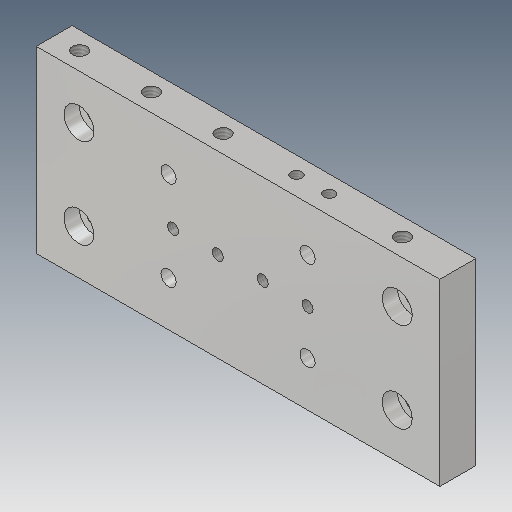
# Autodesk Inventor part: XcolBracket
Saved by Autodesk Inventor 2019 (Build 230136000, 136)
## iProperties
Created: 2018-10-03
Part Number: XcolBracket
Material: Aluminum 6061-AHC
Document SubType Name: Modeling
Designer: LillaHunden
Mass: 74.1972 g
Surface Area: 104.645 cm^2
Volume: 27.4804 cm^3
Density: 2.7 g/cm^3
Appearance: Aluminum - Dark
Author: LillaHunden
Autodesk Inventor part; units mm, degrees
ref_plane "YZ Plane" through (0, 0, 0) normal (1, 0, 0) x (0, 1, 0)
ref_plane "XZ Plane" through (0, 0, 0) normal (0, 1, 0) x (-1, 0, 0)
ref_plane "XY Plane" through (0, 0, 0) normal (0, 0, 1) x (1, 0, 0)
sketch "Sketch1" plane through (0, 0, 0) normal (0, 0, 1) x (1, 0, 0)
  line L0 (22.4756, 17.0801) -> (-67.5244, 17.0801)
  line L1 (-67.5244, 17.0801) -> (-67.5244, -22.9199)
  line L2 (-67.5244, -22.9199) -> (22.4756, -22.9199)
  line L3 (22.4756, -22.9199) -> (22.4756, 17.0801)
  point P0 (0, 0)
  dimension "d0" = 90
  dimension "d53" = 40
  constraints: 8 end point, 2 parallel, 1 horizontal, 1 perpendicular
  measures "d0" distance of L2.end L1.end
  measures "d53" distance of L0.end L1.end
extrude "Extrusion1" add sketch "Sketch1" along normal blind 8
sketch "Sketch2" plane through (0, 0, 8) normal (0, 0, 1) x (1, 0, 0)
  point P0 (12.9756, 7.0801)
  point P1 (12.9756, -12.9199)
  point P2 (-58.0244, 7.0801)
  point P3 (-58.0244, -12.9199)
hole "Hole1" at (12.9756, 7.0801, 8) at (12.9756, -12.9199, 8) at (-58.0244, 7.0801, 8) at (-58.0244, -12.9199, 8) direction (0, 0, -1) diameter 3.4 depth 8 counterbore diameter 6.7 counterbore depth 3.4
sketch "Sketch3" plane through (-67.5244, 17.0801, 0) normal (0, 1, 0) x (1, 0, 0)
  point P0 (61.1484, -12.9831)
  point P1 (53.8516, -12.9831)
  point P2 (61.15, -3.819)
  point P3 (53.85, -3.819)
hole "Hole3" at (-6.376, 17.0801, 12.9831) at (-13.6728, 17.0801, 12.9831) at (-6.3744, 17.0801, 3.819) at (-13.6744, 17.0801, 3.819) direction (0, -1, 0) diameter 2.459 depth 5.4849 tip angle 120 thread size "M3x0.5" class "6H" standard "ISO Metric profile"
sketch "Sketch4" plane through (-67.5244, 17.0801, 0) normal (0, 1, 0) x (1, 0, 0)
  point P0 (37.6646, -15)
  point P1 (37.6646, -4)
  point P2 (21.6646, -4)
  point P3 (5.6646, -4)
  point P4 (77.6646, -4)
hole "Hole5" at (-29.8597, 17.0801, 15) at (-29.8597, 17.0801, 4) at (-45.8597, 17.0801, 4) at (-61.8597, 17.0801, 4) at (10.1403, 17.0801, 4) direction (0, -1, 0) diameter 3.242 depth 5.0229 tip angle 120 thread size "M4x0.7" class "6H" standard "ISO Metric profile"
sketch "Sketch8" plane through (0, 0, 8) normal (0, 0, 1) x (1, 0, 0)
  point P0 (-7.0244, -2.9199)
  point P1 (-17.0244, -2.9199)
  point P2 (-27.0244, -2.9199)
  point P3 (-37.0244, -2.9199)
hole "Hole12" at (-7.0244, -2.9199, 8) at (-17.0244, -2.9199, 8) at (-27.0244, -2.9199, 8) at (-37.0244, -2.9199, 8) direction (0, 0, -1) diameter 2.459 depth 8.4 tip angle 120 thread size "M3x0.5" class "6H" standard "ISO Metric profile"
sketch "Sketch9" plane through (0, 0, 0) normal (0, 0, -1) x (-1, 0, 0)
  point P0 (7.0244, -12.9199)
  point P1 (7.0244, 7.0801)
  point P2 (38.0244, -12.9199)
  point P3 (38.0244, 7.0801)
hole "Hole14" at (-7.0244, -12.9199, 0) at (-7.0244, 7.0801, 0) at (-38.0244, -12.9199, 0) at (-38.0244, 7.0801, 0) direction (0, 0, 1) diameter 3.4 depth 8
body "Solid1"
